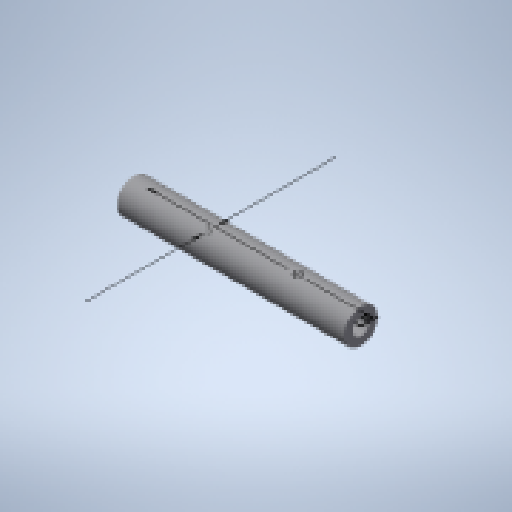
# Autodesk Inventor part: 铜柱
Saved by Autodesk Inventor 2025.2 (Build 292293000, 293)
## iProperties
Created: 2025-09-29
Part Number: 铜柱
Material: 常规
Document SubType Name: Modeling
Designer: BO‘S_SLAVE
Density: 1 g/cm^3
Appearance: 默认
Author: BO‘S_SLAVE
Autodesk Inventor part; units mm, degrees
ref_plane "YZ Plane" through (0, 0, 0) normal (1, 0, 0) x (0, 1, 0)
ref_plane "XZ Plane" through (0, 0, 0) normal (0, 1, 0) x (-1, 0, 0)
ref_plane "XY Plane" through (0, 0, 0) normal (0, 0, 1) x (1, 0, 0)
sketch "草图1" plane through (0, 0, 0) normal (0, 1, 0) x (-1, 0, 0)
  line L0 (0, 0) -> (-40, 0)
  line L1 (-40, 0) -> (-40, -3)
  line L2 (-40, -3) -> (0, -3)
  line L3 (0, -3) -> (0, 0)
  line L4 (0, -1.5) -> (-40, -1.5)
  dimension "d1" = 40
  dimension "d4" = 1.5
  constraints: 10 end point, 2 midpoint, 2 parallel, 1 horizontal, 1 perpendicular
  measures "d1" distance between parallel lines of L1 L3
  measures "d4" distance between parallel lines of L0 L4
revolve "旋转1" add sketch "草图1" angle 360 about axis through (0, 0, 0) along (1, 0, 0)
revolve "旋转2" cut sketch "草图1" angle 360 about axis through (0, 0, 0) along (1, 0, 0) contours L3 L4 L1 L0
